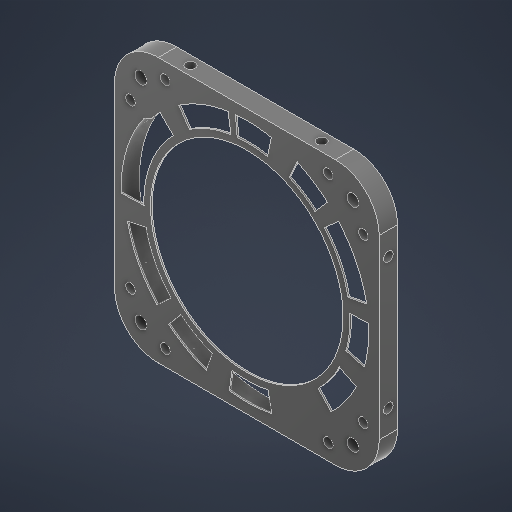
# Autodesk Inventor part: stator_center_01_p
Saved by Autodesk Inventor 2026.1 (Build 301233000, 233)
## iProperties
Created: 2026-04-12
Part Number: stator_center_01_p
Material: PC/ABS Plastic
Document SubType Name: Modeling
Designer: aaron
Density: 1.1 g/cm^3
Appearance: Smooth - White
Author: aaron
Autodesk Inventor part; units mm, degrees
ref_plane "YZ Plane" through (0, 0, 0) normal (1, 0, 0) x (0, 1, 0)
ref_plane "XZ Plane" through (0, 0, 0) normal (0, 1, 0) x (-1, 0, 0)
ref_plane "XY Plane" through (0, 0, 0) normal (0, 0, 1) x (1, 0, 0)
sketch "Sketch1" plane through (0, 0, 0) normal (0, 0, 1) x (1, 0, 0)
  circle A0 centre (0, 0) radius 57.5
  circle A1 centre (0, 0) radius 60.5
  line L0 (-40.5, 60.5) -> (40.5, 60.5)
  line L1 (60.5, 40.5) -> (60.5, -40.5)
  line L2 (40.5, -60.5) -> (-40.5, -60.5)
  line L3 (-60.5, -40.5) -> (-60.5, 40.5)
  arc A2 (-40.5, 60.5) -> (-60.5, 40.5) centre (-40.5, 40.5) ccw
  arc A3 (60.5, 40.5) -> (40.5, 60.5) centre (40.5, 40.5) ccw
  arc A4 (40.5, -60.5) -> (60.5, -40.5) centre (40.5, -40.5) ccw
  arc A5 (-60.5, -40.5) -> (-40.5, -60.5) centre (-40.5, -40.5) ccw
  dimension "d0" = 115
  dimension "d1" = 121
  dimension "d2" = 20
  constraints: 12 tangent, 8 end point, 8 point on circle, 6 centre point, 3 equal radius, 2 coincident, 2 parallel, 1 horizontal, 1 perpendicular
  measures "d0" diameter of A0
  measures "d1" diameter of A1
  measures "d2" radius of A2
extrude "Extrusion1" add sketch "Sketch1" along normal blind 7.7
sketch "Sketch3" plane through (0, 0, 7.7) normal (0, 0, 1) x (1, 0, 0)
  circle A0 centre (-48.4934, -48.5066) radius 2.65 projected
  circle A1 centre (-37.2752, -53.25) radius 2.15 projected
  circle A2 centre (-53.2398, -37.2897) radius 2.15 projected
  circle A3 centre (-53.25, 37.2752) radius 2.15 projected
  circle A4 centre (-48.5066, 48.4934) radius 2.65 projected
  circle A5 centre (-37.2897, 53.2398) radius 2.15 projected
  circle A6 centre (53.2398, 37.2897) radius 2.15 projected
  circle A7 centre (48.4934, 48.5066) radius 2.65 projected
  circle A8 centre (37.2752, 53.25) radius 2.15 projected
  circle A9 centre (53.25, -37.2752) radius 2.15 projected
  circle A10 centre (48.5066, -48.4934) radius 2.65 projected
  circle A11 centre (37.2897, -53.2398) radius 2.15 projected
  point P0 (0, 0)
extrude "Extrusion3" cut sketch "Sketch3" against normal through all
sketch "Sketch4" plane through (0, 0, 7.7) normal (0, 0, 1) x (1, 0, 0)
  circle A0 centre (0, 0) radius 29 projected
  line L0 (9.6493, -46.097) -> (11.4281, -54.5943) projected
  arc A1 (-7.99, -55.2023) -> (11.4281, -54.5943) centre (0, 0) ccw projected
  line L1 (-7.99, -55.2023) -> (-6.7464, -46.6104) projected
  arc A2 (-6.7464, -46.6104) -> (9.6493, -46.097) centre (0, 0) ccw projected
  line L2 (-26.2539, 39.0996) -> (-31.0934, 46.307) projected
  arc A3 (-8.5912, 55.112) -> (-31.0934, 46.307) centre (0, 0) ccw projected
  line L3 (-8.5912, 55.112) -> (-7.254, 46.5341) projected
  arc A4 (-7.254, 46.5341) -> (-26.2539, 39.0996) centre (0, 0) ccw projected
  line L4 (53.6989, -15.0854) -> (45.341, -12.7375) projected
  arc A5 (45.341, -12.7375) -> (47.0109, 2.8322) centre (0, 0) ccw projected
  line L5 (47.0109, 2.8322) -> (55.6766, 3.3542) projected
  arc A6 (53.6989, -15.0854) -> (55.6766, 3.3542) centre (0, 0) ccw projected
  line L6 (54.7773, 10.5158) -> (46.2516, 8.8791) projected
  arc A7 (46.2516, 8.8791) -> (35.4257, 31.0334) centre (0, 0) ccw projected
  line L7 (35.4257, 31.0334) -> (41.9558, 36.7539) projected
  arc A8 (54.7773, 10.5158) -> (41.9558, 36.7539) centre (0, 0) ccw projected
  line L8 (-15.7851, -44.372) -> (-18.6949, -52.5513) projected
  arc A9 (-35.715, -42.8436) -> (-18.6949, -52.5513) centre (0, 0) ccw projected
  line L9 (-35.715, -42.8436) -> (-30.1562, -36.1753) projected
  arc A10 (-30.1562, -36.1753) -> (-15.7851, -44.372) centre (0, 0) ccw projected
  line L10 (11.2228, 54.6369) -> (9.4761, 46.133) projected
  arc A11 (9.4761, 46.133) -> (-4.3919, 46.8909) centre (0, 0) ccw projected
  line L11 (-4.3919, 46.8909) -> (-5.2015, 55.5345) projected
  arc A12 (11.2228, 54.6369) -> (-5.2015, 55.5345) centre (0, 0) ccw projected
  line L12 (38.5468, -40.3148) -> (32.5472, -34.04) projected
  arc A13 (32.5472, -34.04) -> (42.2602, -20.7876) centre (0, 0) ccw projected
  line L13 (42.2602, -20.7876) -> (50.0502, -24.6195) projected
  arc A14 (38.5468, -40.3148) -> (50.0502, -24.6195) centre (0, 0) ccw projected
  line L14 (36.8913, 41.835) -> (31.1494, 35.3237) projected
  arc A15 (31.1494, 35.3237) -> (19.437, 42.8982) centre (0, 0) ccw projected
  line L15 (19.437, 42.8982) -> (23.0199, 50.8058) projected
  arc A16 (36.8913, 41.835) -> (23.0199, 50.8058) centre (0, 0) ccw projected
  line L16 (-34.6849, -31.8592) -> (-41.0785, -37.7319) projected
  arc A17 (-54.5943, -11.4281) -> (-41.0785, -37.7319) centre (0, 0) ccw projected
  line L17 (-54.5943, -11.4281) -> (-46.097, -9.6493) projected
  arc A18 (-46.097, -9.6493) -> (-34.6849, -31.8592) centre (0, 0) ccw projected
  circle A19 centre (37.2752, 53.25) radius 2.15 projected
  circle A20 centre (16.4961, 28.5811) radius 1.25 projected
  circle A21 centre (-37.2752, -53.25) radius 2.15 projected
  circle A22 centre (-37.2897, 53.2398) radius 2.15 projected
  circle A23 centre (48.5066, -48.4934) radius 2.65 projected
  circle A24 centre (-48.4934, -48.5066) radius 2.65 projected
  circle A25 centre (-53.25, 37.2752) radius 2.15 projected
  circle A26 centre (-53.2398, -37.2897) radius 2.15 projected
  circle A27 centre (16.5039, -28.5766) radius 1.25 projected
  circle A28 centre (53.2398, 37.2897) radius 2.15 projected
  circle A29 centre (53.25, -37.2752) radius 2.15 projected
  circle A30 centre (-16.4961, -28.5811) radius 1.25 projected
  circle A31 centre (-16.5039, 28.5766) radius 1.25 projected
  circle A32 centre (48.4934, 48.5066) radius 2.65 projected
  circle A33 centre (-48.5066, 48.4934) radius 2.65 projected
  circle A34 centre (-33, -0.0045) radius 1.25 projected
  circle A35 centre (37.2897, -53.2398) radius 2.15 projected
  circle A36 centre (33, 0.0045) radius 1.25 projected
  line L18 (-59.5162, 33.2815) -> (-60.5047, 34.4337) projected
  line L19 (-59.5162, 33.2815) -> (-50.1662, 31.842) projected
  line L20 (-43.8555, 34.4649) -> (-50.1662, 31.842) projected
  arc A37 (-39.7545, 39.1244) -> (-43.8555, 34.4649) centre (0, 0) ccw projected
  line L21 (-39.7545, 39.1244) -> (-33.5669, 33.0349) projected
  arc A38 (-33.5669, 33.0349) -> (-47.0756, -1.3908) centre (0, 0) ccw projected
  line L22 (-47.0756, -1.3908) -> (-55.7533, -1.6472) projected
  line L23 (-55.7533, -1.6472) -> (-59.4998, -1.6477) projected
  line L24 (-60.4996, -2.6478) -> (-59.4998, -1.6477) projected
  line L25 (-60.4996, -2.6478) -> (-60.4945, -40.5083) projected
  arc A39 (-60.4945, -40.5083) -> (-40.4917, -60.5055) centre (-40.4945, -40.5055) ccw projected
  line L26 (-40.4917, -60.5055) -> (40.5083, -60.4945) projected
  arc A40 (40.5083, -60.4945) -> (60.5055, -40.4917) centre (40.5055, -40.4945) ccw projected
  line L27 (60.5055, -40.4917) -> (60.4945, 40.5083) projected
  arc A41 (60.4945, 40.5083) -> (40.4917, 60.5055) centre (40.4945, 40.5055) ccw projected
  line L28 (40.4917, 60.5055) -> (-40.5083, 60.4945) projected
  arc A42 (-40.5083, 60.4945) -> (-60.5055, 40.4917) centre (-40.5055, 40.4945) ccw projected
  line L29 (-60.5055, 40.4917) -> (-60.5047, 34.4337) projected
  circle A43 centre (-53.2398, -37.2897) radius 2.15 projected
  circle A44 centre (53.2398, 37.2897) radius 2.15 projected
  circle A45 centre (48.5066, -48.4934) radius 2.65 projected
  circle A46 centre (37.2897, -53.2398) radius 2.15 projected
  circle A47 centre (-37.2897, 53.2398) radius 2.15 projected
  circle A48 centre (-48.4934, -48.5066) radius 2.65 projected
  circle A49 centre (-53.25, 37.2752) radius 2.15 projected
  circle A50 centre (48.4934, 48.5066) radius 2.65 projected
  circle A51 centre (53.25, -37.2752) radius 2.15 projected
  circle A52 centre (37.2752, 53.25) radius 2.15 projected
  circle A53 centre (-48.5066, 48.4934) radius 2.65 projected
  circle A54 centre (-37.2752, -53.25) radius 2.15 projected
  line L30 (-60.5, 40.5) -> (-60.5, -40.5) projected
  arc A55 (-60.5, -40.5) -> (-40.5, -60.5) centre (-40.5, -40.5) ccw projected
  line L31 (-40.5, -60.5) -> (40.5, -60.5) projected
  arc A56 (40.5, -60.5) -> (60.5, -40.5) centre (40.5, -40.5) ccw projected
  line L32 (60.5, -40.5) -> (60.5, 40.5) projected
  arc A57 (60.5, 40.5) -> (40.5, 60.5) centre (40.5, 40.5) ccw projected
  line L33 (40.5, 60.5) -> (-40.5, 60.5) projected
  arc A58 (-40.5, 60.5) -> (-60.5, 40.5) centre (-40.5, 40.5) ccw projected
  circle A59 centre (0, 0) radius 57.5 projected
  point P0 (-54.6384, -54.6459)
  point P1 (0.0041, -60.5)
  point P2 (54.6459, -54.6384)
  point P3 (60.5, 0.0041)
  point P4 (54.6384, 54.6459)
  point P5 (-0.0041, 60.5)
  point P6 (-54.6459, 54.6384)
  point P7 (-60.5, 34.4282)
  point P8 (-57.4764, -1.6474)
  point P9 (-46.9668, 33.1718)
extrude "Extrusion4" add sketch "Sketch4" along normal blind 0.7 contours L19 L20 A59 L23 L24 L30 L18 | L18 L30 A58 A42 L28 L33 A57 A41 L27 L32 A56 A40 L26 L31 A55 A39 L25 L24 L23 A59 L20 L19 | L25 A39 A55 L30 | A59 L23 L22 A38 L21 A37 L20 | A58 L33 L28 A42 | L26 A40 A56 L31 | A57 L32 L27 A41 picked at (17.5819, -42.3508)
sketch "Sketch5" plane through (0, 0, 8.4) normal (0, 0, 1) x (1, 0, 0)
  circle A0 centre (-33, -0.0045) radius 1.25 projected
  circle A1 centre (-33, -0.0045) radius 1.75
  circle A2 centre (-16.4961, -28.5811) radius 1.75
  circle A3 centre (16.5039, -28.5766) radius 1.75
  circle A4 centre (33, 0.0045) radius 1.75
  circle A5 centre (16.4961, 28.5811) radius 1.75
  circle A6 centre (-16.5039, 28.5766) radius 1.75
  point P0 (0, 0)
  dimension "d30" = 3.5
  dimension "d33" = 360
  constraints: 6 centre point, 1 coincident, 13 other
  measures "d30" diameter of A1
extrude "Extrusion5" cut sketch "Sketch5" against normal through all contours A0 | A1 | A2 | A3 | A4 | A5 | A6
sketch "Sketch6" plane through (0, 0, 7.7) normal (0, 0, -1) x (-1, 0, 0)
  circle A0 centre (0, 0) radius 35
  circle A1 centre (-33, 0.0045) radius 1.75 projected
  circle A2 centre (33, -0.0045) radius 1.75 projected
  circle A3 centre (-16.5039, -28.5766) radius 1.75 projected
  circle A4 centre (-16.4961, 28.5811) radius 1.75 projected
  circle A5 centre (16.5039, 28.5766) radius 1.75 projected
  circle A6 centre (16.4961, -28.5811) radius 1.75 projected
  circle A7 centre (0, 0) radius 29 projected
  line L0 (7.99, -55.2023) -> (6.7464, -46.6104) projected
  arc A8 (-11.4281, -54.5943) -> (7.99, -55.2023) centre (0, 0) ccw projected
  line L1 (-9.6493, -46.097) -> (-11.4281, -54.5943) projected
  arc A9 (-9.6493, -46.097) -> (6.7464, -46.6104) centre (0, 0) ccw projected
  line L2 (8.5912, 55.112) -> (7.254, 46.5341) projected
  arc A10 (31.0934, 46.307) -> (8.5912, 55.112) centre (0, 0) ccw projected
  line L3 (26.2539, 39.0996) -> (31.0934, 46.307) projected
  arc A11 (26.2539, 39.0996) -> (7.254, 46.5341) centre (0, 0) ccw projected
  line L4 (-53.6989, -15.0854) -> (-45.341, -12.7375) projected
  arc A12 (-55.6766, 3.3542) -> (-53.6989, -15.0854) centre (0, 0) ccw projected
  line L5 (-47.0109, 2.8322) -> (-55.6766, 3.3542) projected
  arc A13 (-47.0109, 2.8322) -> (-45.341, -12.7375) centre (0, 0) ccw projected
  line L6 (-54.7773, 10.5158) -> (-46.2516, 8.8791) projected
  arc A14 (-41.9558, 36.7539) -> (-54.7773, 10.5158) centre (0, 0) ccw projected
  line L7 (-35.4257, 31.0334) -> (-41.9558, 36.7539) projected
  arc A15 (-35.4257, 31.0334) -> (-46.2516, 8.8791) centre (0, 0) ccw projected
  line L8 (35.715, -42.8436) -> (30.1562, -36.1753) projected
  arc A16 (18.6949, -52.5513) -> (35.715, -42.8436) centre (0, 0) ccw projected
  line L9 (15.7851, -44.372) -> (18.6949, -52.5513) projected
  arc A17 (15.7851, -44.372) -> (30.1562, -36.1753) centre (0, 0) ccw projected
  line L10 (-11.2228, 54.6369) -> (-9.4761, 46.133) projected
  arc A18 (5.2015, 55.5345) -> (-11.2228, 54.6369) centre (0, 0) ccw projected
  line L11 (4.3919, 46.8909) -> (5.2015, 55.5345) projected
  arc A19 (4.3919, 46.8909) -> (-9.4761, 46.133) centre (0, 0) ccw projected
  line L12 (-38.5468, -40.3148) -> (-32.5472, -34.04) projected
  arc A20 (-50.0502, -24.6195) -> (-38.5468, -40.3148) centre (0, 0) ccw projected
  line L13 (-42.2602, -20.7876) -> (-50.0502, -24.6195) projected
  arc A21 (-42.2602, -20.7876) -> (-32.5472, -34.04) centre (0, 0) ccw projected
  line L14 (-36.8913, 41.835) -> (-31.1494, 35.3237) projected
  arc A22 (-23.0199, 50.8058) -> (-36.8913, 41.835) centre (0, 0) ccw projected
  line L15 (-19.437, 42.8982) -> (-23.0199, 50.8058) projected
  arc A23 (-19.437, 42.8982) -> (-31.1494, 35.3237) centre (0, 0) ccw projected
  line L16 (54.5943, -11.4281) -> (46.097, -9.6493) projected
  arc A24 (41.0785, -37.7319) -> (54.5943, -11.4281) centre (0, 0) ccw projected
  line L17 (34.6849, -31.8592) -> (41.0785, -37.7319) projected
  arc A25 (34.6849, -31.8592) -> (46.097, -9.6493) centre (0, 0) ccw projected
  arc A26 (46.9668, 33.1718) -> (57.4764, -1.6474) centre (0, 0) ccw projected
  line L18 (55.7533, -1.6472) -> (57.4764, -1.6474) projected
  line L19 (47.0756, -1.3908) -> (55.7533, -1.6472) projected
  arc A27 (47.0756, -1.3908) -> (33.5669, 33.0349) centre (0, 0) ccw projected
  line L20 (39.7545, 39.1244) -> (33.5669, 33.0349) projected
  arc A28 (43.8555, 34.4649) -> (39.7545, 39.1244) centre (0, 0) ccw projected
  line L21 (46.9668, 33.1718) -> (43.8555, 34.4649) projected
  dimension "d37" = 70
  constraints: 1 centre point, 1 coincident
  measures "d37" diameter of A0
extrude "Extrusion6" add sketch "Sketch6" along normal blind 0.5 contours A0
sketch "Sketch8" plane through (0, 0, 8.4) normal (0, 0, 1) x (1, 0, 0)
  circle A0 centre (0, 0) radius 44
  dimension "d46" = 88
  constraints: 1 centre point, 1 coincident
  measures "d46" diameter of A0
extrude "Extrusion8" cut sketch "Sketch8" against normal through all
sketch "Sketch9" plane through (-40.5, 60.5, 0) normal (0, 1, 0) x (1, 0, 0)
  circle A0 centre (10.5, -4.15) radius 2.15
  line L0 (101, 0) -> (101, -8.4) projected
  line L1 (-20, 0) -> (-20, -8.4) projected
  line L2 (81, -8.4) -> (0, -8.4) projected
  circle A1 centre (70.5, -4.15) radius 2.15
  point P0 (40.5, 0)
  dimension "d49" = 4.3
  dimension "d50" = 121
  dimension "d51" = 4.25
  dimension "d52" = 30.5
  dimension "d55" = 60
  constraints: 2 centre point, 1 horizontal, 2 other
  measures "d49" diameter of A0
  measures "d50" distance between parallel lines of L0 L1
  measures "d51" distance from line of L2 A0.centre
  measures "d52" distance from line of L1 A0.centre
  measures "d55" distance of A0.centre A1.centre
extrude "Extrusion9" cut sketch "Sketch9" against normal blind 10
sketch "Sketch10" plane through (-40.5, -60.5, 0) normal (0, -1, 0) x (1, 0, 0)
  circle A0 centre (10.5, 4.15) radius 2.15 projected
  circle A1 centre (70.5, 4.15) radius 2.15 projected
  point P0 (40.5, 0)
extrude "Extrusion10" cut sketch "Sketch10" against normal blind 10
sketch "Sketch11" plane through (60.5, -40.5, 0) normal (1, 0, 0) x (0, 0, -1)
  circle A0 centre (-4.15, 10.5) radius 2.15
  line L0 (0, 101) -> (-8.4, 101) projected
  line L1 (0, -20) -> (-8.4, -20) projected
  line L2 (-8.4, 0) -> (-8.4, -20) projected
  circle A1 centre (-4.15, 70.5) radius 2.15
  point P0 (0, 40.5)
  dimension "d64" = 4.3
  dimension "d65" = 121
  dimension "d66" = 4.25
  dimension "d67" = 30.5
  dimension "d70" = 60
  constraints: 2 centre point, 1 vertical, 2 other
  measures "d64" diameter of A0
  measures "d65" distance between parallel lines of L0 L1
  measures "d66" distance from line of L2 A0.centre
  measures "d67" distance from line of L1 A0.centre
  measures "d70" distance of A0.centre A1.centre
extrude "Extrusion11" cut sketch "Sketch11" against normal blind 10
sketch "Sketch12" plane through (-60.5, -40.5, 0) normal (-1, 0, 0) x (0, 0, 1)
  circle A0 centre (4.15, 70.5) radius 2.15 projected
  circle A1 centre (4.15, 10.5) radius 2.15 projected
  point P0 (0, 40.5)
extrude "Extrusion12" cut sketch "Sketch12" against normal blind 10
body "Solid1"
